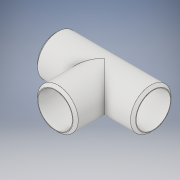
# Autodesk Inventor part: Tee 1.25 IN D
Saved by Autodesk Inventor 2019 (Build 230136000, 136)
## iProperties
Created: 2019-07-05
Part Number: Tee 1.25 IN D
Material: PVC-Piping
Document SubType Name: Modeling
Designer: J. LENDI
Mass: 117.33 g
Surface Area: 446.191 cm^2
Volume: 83.8073 cm^3
Density: 1.4 g/cm^3
Appearance: Smooth - White
Author: J. LENDI
Autodesk Inventor part; units mm, degrees
ref_plane "YZ Plane" through (0, 0, 0) normal (1, 0, 0) x (0, 1, 0)
ref_plane "XZ Plane" through (0, 0, 0) normal (0, 1, 0) x (-1, 0, 0)
sketch "Sketch1" plane through (0, 0, 0) normal (1, 0, 0) x (0, 1, 0)
  circle A0 centre (0, 0) radius 21.082
  circle A1 centre (0, 0) radius 25.0063
  dimension "d0" = 42.164
  dimension "d1" = 50.0126
  constraints: 2 centre point, 2 coincident
  measures "d0" diameter of A0
  measures "d1" diameter of A1
extrude "Extrusion1" add sketch "Sketch1" along normal mid plane 120.5992
ref_plane "Work Plane1" through (0, 0, 60.3123) normal (0, 0, 1) x (1, 0, 0)
sketch "Sketch2" plane through (0, 0, 60.3123) normal (0, 0, 1) x (1, 0, 0)
  circle A0 centre (0, 0) radius 25.0063
  circle A1 centre (0, 0) radius 21.082
  dimension "d5" = 50.0126
  dimension "d6" = 42.164
  constraints: 2 centre point, 2 coincident
  measures "d5" diameter of A0
  measures "d6" diameter of A1
extrude "Extrusion2" add sketch "Sketch2" against normal up to next
sketch "Sketch3" plane through (0, 0, 60.3123) normal (0, 0, 1) x (1, 0, 0)
  circle A0 centre (0, 0) radius 21.082 projected
extrude "Extrusion3" cut sketch "Sketch3" against normal up to next
chamfer "Chamfer1" distance 3.175 angle 45 3 edges at (-60.2996, -25.0063, 0) (-25.0063, 0, 60.3123) (60.2996, -25.0063, 0)
body "Solid1"
